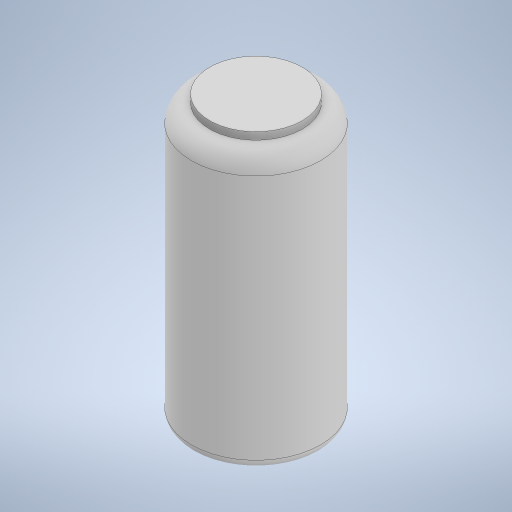
# Autodesk Inventor part: flask
Saved by Autodesk Inventor 2023 (Build 270158000, 158)
## iProperties
Created: 2023-08-31
Part Number: flask
Material: Generic
Document SubType Name: Modeling
Designer: 1908174
Density: 1 g/cm^3
Appearance: Default
Author: 1908174
Autodesk Inventor part; units mm, degrees
ref_plane "YZ Plane" through (0, 0, 0) normal (1, 0, 0) x (0, 1, 0)
ref_plane "XZ Plane" through (0, 0, 0) normal (0, 1, 0) x (-1, 0, 0)
ref_plane "XY Plane" through (0, 0, 0) normal (0, 0, 1) x (1, 0, 0)
sketch "Sketch1" plane through (0, 0, 0) normal (0, 1, 0) x (-1, 0, 0)
  circle A0 centre (0, 0) radius 44.9961
  dimension "d0" = 89.9922
  constraints: 1 centre point, 1 coincident
  measures "d0" diameter of A0
extrude "Extrusion1" add sketch "Sketch1" along normal blind 190.5
fillet "Fillet1" radius 12.7 1 edges at (44.9961, 190.5, 0)
sketch "Sketch3" plane through (0, 190.5, 0) normal (0, 1, 0) x (1, 0, 0)
  circle A0 centre (0, 0) radius 32.2961
  constraints: 1 centre point, 1 coincident
extrude "Extrusion2" add sketch "Sketch3" along normal blind 5.08
fillet "Fillet2" radius 6.35 1 edges at (44.9961, 0, 0)
body "Solid1"
